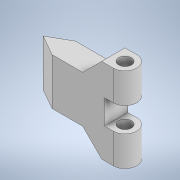
# Autodesk Inventor part: short_link_v3
Saved by Autodesk Inventor 2022 (Build 260153000, 153)
## iProperties
Created: 2022-05-21
Part Number: short_link_v3
Material: Generic
Document SubType Name: Modeling
Designer: kylem
Density: 1 g/cm^3
Appearance: Default
Author: kylem
Autodesk Inventor part; units mm, degrees
ref_plane "YZ Plane" through (0, 0, 0) normal (1, 0, 0) x (0, 1, 0)
sketch "Sketch1" plane through (0, 0, 0) normal (0, 1, 0) x (-1, 0, 0)
  line L0 (0, 0) -> (18, 0)
  line L1 (18, 0) -> (18, -4)
  line L2 (18, -4) -> (0, -4)
  line L3 (0, -4) -> (0, 0)
  line L4 (18, -2) -> (16, -2)
  line L5 (9, -4) -> (9, -3)
  circle A0 centre (16, -2) radius 1.1
  circle A1 centre (2, -2) radius 1.1
  dimension "d0" = 18
  dimension "d1" = 4
  dimension "d2" = 2
  dimension "d3" = 2.2
  constraints: 12 end point, 2 centre point, 2 horizontal, 2 midpoint, 2 parallel, 1 coincident, 1 perpendicular, 1 symmetric about line, 1 vertical, 1 other
  measures "d0" distance of L1.end L2.end
  measures "d1" distance of L0.end L1.end
  measures "d2" distance of L4.start L4.end
  measures "d3" diameter of A0
extrude "Extrusion1" add sketch "Sketch1" along normal blind 8 contours A0 | L0 L1 L2 L3 | A1
sketch "Sketch2" plane through (0, 0, -4) normal (0, 0, -1) x (-1, 0, 0)
  line L0 (18, 0) -> (18, 8) projected
  line L1 (18, 8) -> (18, 6.1)
  line L2 (18, 0) -> (0, 0) projected
  line L3 (18, 0) -> (18, 1.9)
  line L4 (18, 6.1) -> (14.5, 6.1)
  line L5 (14.5, 6.1) -> (14.5, 1.9)
  line L6 (14.5, 1.9) -> (18, 1.9)
  line L7 (18, 1.9) -> (18, 6.1)
  dimension "d6" = 1.9
  dimension "d7" = 1.9
  dimension "d8" = 3.5
  constraints: 12 end point, 2 parallel, 2 point on line, 1 horizontal, 1 perpendicular
  measures "d6" distance of L0.end L1.end
  measures "d7" distance of L0.start L3.end
  measures "d8" distance of L6.end L5.end
extrude "Extrusion2" cut sketch "Sketch2" against normal blind 8
ref_plane "Work Plane1" through (-9, 0, 0) normal (1, 0, 0) x (0, 0, -1)
mirror "Mirror1" about plane through (-9, 0, 0) normal (1, 0, 0) of "Extrusion2"
extrude "Extrusion3" cut sketch "Sketch1" along normal blind 8 contours A0 | A1
sketch "Sketch4" plane through (0, 8, 0) normal (0, 1, 0) x (1, 0, 0)
  line L0 (-18, 0) -> (0, 0) projected
  line L1 (0, 0) -> (-4, 0)
  line L2 (-4, 0) -> (-4, 4)
  line L3 (-4, 4) -> (0, 4)
  line L4 (0, 4) -> (0, 0)
  circle A0 centre (-2, 2) radius 1.1 projected
  circle A1 centre (-2, 2) radius 1.1
  dimension "d14" = 4
  dimension "d15" = 4
  dimension "d16" = 2.2
  constraints: 8 end point, 2 parallel, 1 centre point, 1 coincident, 1 horizontal, 1 perpendicular
  measures "d14" distance of L2.end L3.end
  measures "d15" distance of L1.end L2.end
  measures "d16" diameter of A1
extrude "Extrusion4" add sketch "Sketch4" along normal blind 3.25
ref_plane "Work Plane2" through (-3.5, 4, 0) normal (0, 1, 0) x (1, 0, 0)
mirror "Mirror2" about plane through (-3.5, 4, 0) normal (0, 1, 0) of "Extrusion4"
fillet "Fillet2" radius 2 8 edges at (0, 8.675, -4) (0, -0.675, -4) (0, -0.675, 0) (0, 8.675, 0) (-18, 7.05, -4) (-18, 0.95, -4) (-18, 7.05, 0) (-18, 0.95, 0)
chamfer "Chamfer1" distance 3.25 angle 45 2 edges at (-4, 8, -2) (-4, 0, -2)
sketch "Sketch5" plane through (-14.5, 1.9, 0) normal (0, 0, 1) x (1, 0, 0)
  line L0 (0, 0) -> (-1.5, 0) projected
  line L1 (0, 0) -> (-4.1729, 0)
  line L2 (-4.1729, 0) -> (-4.1729, 7.3414)
  line L3 (-4.1729, 7.3414) -> (0, 7.3414)
  line L4 (0, 7.3414) -> (0, 0)
  line L5 (0, 0) -> (-4.2733, 0)
  line L6 (-4.2733, 0) -> (-4.2733, -4.4882)
  line L7 (-4.2733, -4.4882) -> (0, -4.4882)
  line L8 (0, -4.4882) -> (0, 0)
  point P0 (14.5, -1.9)
  constraints: 16 end point, 4 parallel, 2 horizontal, 2 perpendicular
extrude "Extrusion5" cut sketch "Sketch5" against normal blind 10
sketch "Sketch6" plane through (0, 0, 0) normal (0, -1, 0) x (1, 0, 0)
  line L0 (-14.5, 0) -> (-14.5, -4) projected
  line L1 (-14.5, -2) -> (-16, -2)
  line L2 (-14.5, 0) -> (-7.25, 0) projected
  line L3 (-7.25, -4) -> (-14.5, -4) projected
  line L4 (-14.5, 0) -> (-12.5, 0)
  line L5 (-12.5, 0) -> (-12.5, -4)
  line L6 (-12.5, -4) -> (-14.5, -4)
  line L7 (-14.5, -4) -> (-14.5, 0)
  point P0 (0, 0)
  dimension "d25" = 1.5
  dimension "d26" = 2
  constraints: 10 end point, 2 horizontal, 2 parallel, 1 midpoint, 1 perpendicular, 1 point on line
  measures "d25" distance of L1.start L1.end
  measures "d26" distance of L5.end L6.end
extrude "Extrusion6" cut sketch "Sketch6" against normal blind 10
sketch "Sketch7" plane through (0, 0, 0) normal (0, -1, 0) x (1, 0, 0)
  line L0 (-12.5, 0) -> (-12.5, -4) projected
  line L1 (-12.5, -2) -> (-16, -2)
  line L2 (-12.5, 0) -> (-7.25, 0) projected
  line L3 (-16, -2) -> (-12.5, 0)
  line L4 (-7.25, -4) -> (-12.5, -4) projected
  line L5 (-12.5, 0) -> (-12.5, -4)
  line L6 (-12.5, -4) -> (-16, -2)
  point P0 (0, 0)
  dimension "d29" = 3.5
  constraints: 8 end point, 1 horizontal, 1 midpoint, 1 perpendicular
  measures "d29" distance of L1.start L1.end
extrude "Extrusion7" add sketch "Sketch7" against normal blind 8
body "Solid1"
